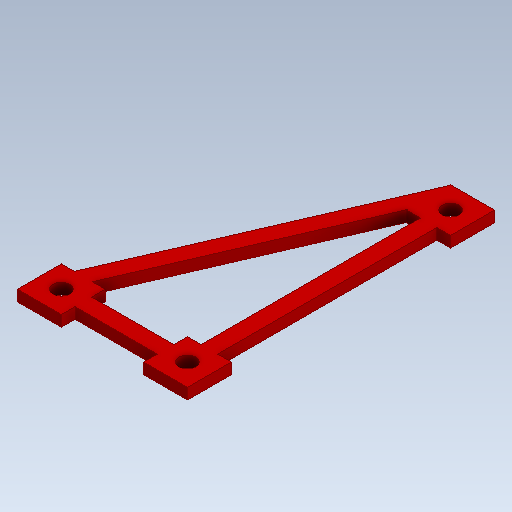
# Autodesk Inventor part: HexServoCoverV2
Saved by Autodesk Inventor 2020 (Build 240168000, 168)
## iProperties
Created: 2023-12-31
Part Number: HexServoCoverV2
Material: PETG
Document SubType Name: Modeling
Designer: smz3rm
Density: 1 g/cm^3
Appearance: Generic
Author: smz3rm
Autodesk Inventor part; units mm, degrees
ref_plane "YZ Plane" through (0, 0, 0) normal (1, 0, 0) x (0, 1, 0)
ref_plane "XZ Plane" through (0, 0, 0) normal (0, 1, 0) x (-1, 0, 0)
ref_plane "XY Plane" through (0, 0, 0) normal (0, 0, 1) x (1, 0, 0)
derived "HexBodyV2.ipt"
sketch "Sketch14" plane through (-59, -12, 62.4426) normal (0, 1, 0) x (1, 0, 0)
  line L0 (7, 63.7574) -> (48, 63.7574)
  line L1 (48, 63.7574) -> (48, 23.7574)
  line L2 (48, 23.7574) -> (7, 23.7574)
  line L3 (7, 23.7574) -> (7, 63.7574)
  line L4 (51, 66.7574) -> (4.5, 66.7574)
  line L5 (4.5, 20.7574) -> (51, 20.7574)
  line L6 (51, 20.7574) -> (51, 66.7574)
  line L7 (40, 66.7574) -> (40, 20.7574)
  line L8 (35, 66.7574) -> (35, 20.7574)
  line L9 (7, 63.7574) -> (35, 63.7574)
  line L10 (4, 43.7574) -> (51, 43.7574)
  line L11 (15.5, 66.7574) -> (15.5, 63.7574)
  line L12 (11, 66.7574) -> (11, 63.7574)
  line L13 (48, 53.7574) -> (54, 53.7574)
  line L14 (54, 53.7574) -> (59, 53.7574)
  line L15 (59, 167.4426) -> (59, -42.5574)
  line L16 (48, 68.5926) -> (48, 66.2926)
  line L17 (4.5, 66.7574) -> (4, 66.7574)
  line L18 (4, 8.833) -> (4, 87.1926)
  line L19 (4, 0.833) -> (4, 124.0523)
  line L20 (4.5, 20.7574) -> (4, 20.7574)
  line L21 (35, 23.7574) -> (27, 23.7574)
  line L22 (27, 23.7574) -> (27, 15.7574)
  line L23 (27, 15.7574) -> (35, 15.7574)
  line L24 (35, 15.7574) -> (35, 23.7574)
  line L25 (27, 63.7574) -> (27, 71.7574)
  line L26 (27, 71.7574) -> (35, 71.7574)
  line L27 (35, 71.7574) -> (35, 63.7574)
  line L28 (12, 23.7574) -> (4, 23.7574)
  line L29 (4, 23.7574) -> (4, 15.7574)
  line L30 (4, 15.7574) -> (12, 15.7574)
  line L31 (12, 15.7574) -> (12, 23.7574)
  line L32 (42, 63.8053) -> (42, 88.0017)
  line L33 (42, 66.7574) -> (42, 63.7574)
  line L34 (48, 63.7574) -> (48, 63.8053)
  line L35 (48, 63.8053) -> (42, 63.8053)
  line L36 (48, 63.7574) -> (48, 63.7574)
  line L37 (48, 63.7574) -> (48, 63.8053)
  point P0 (59, 62.4426)
  point P1 (34.5, 20.5208)
  point P2 (41, 65.8053)
  point P3 (11, 63.7574)
  point P4 (15.5, 63.7574)
  point P5 (48, 67.4426)
  point P6 (48, 43.7574)
  point P7 (40, 23.7574)
  point P8 (27, 66.7574)
  point P9 (35, 66.7574)
  point P10 (35, 20.7574)
  point P11 (27, 20.7574)
  point P12 (12, 20.7574)
  point P13 (40, 63.7574)
  point P14 (42, 63.8053)
  point P15 (42, 63.8053)
sketch "Sketch2" plane through (0, 0, 0) normal (0, 1, 0) x (-1, 0, 0)
  line L0 (32, -1.3148) -> (32, -9.3148) projected
  line L1 (32, -9.3148) -> (24, -9.3148) projected
  line L2 (24, -9.3148) -> (24, -1.3148) projected
  line L3 (32, 38.6852) -> (32, 46.6852) projected
  line L4 (24, 46.6852) -> (24, 38.6852) projected
  line L5 (32, 46.6852) -> (24, 46.6852) projected
  line L6 (55, 46.6852) -> (47, 46.6852) projected
  line L7 (47, 46.6852) -> (47, 38.6852) projected
  line L8 (47, 38.6852) -> (55, 38.6852) projected
  line L9 (55, 38.6852) -> (55, 46.6852)
  line L10 (32, 38.6852) -> (24, 38.6852)
  line L11 (32, -1.3148) -> (24, -1.3148)
  line L12 (32, -9.3148) -> (24, -1.3148)
  line L13 (32, 38.6852) -> (24, 46.6852)
  line L14 (55, 38.6852) -> (47, 46.6852)
  circle A0 centre (28, -5.3148) radius 1.55
  circle A1 centre (28, 42.6852) radius 1.55
  circle A2 centre (51, 42.6852) radius 1.55
  line L15 (47, 41.1852) -> (32, 41.1852)
  line L16 (32, 41.1852) -> (32, 44.1852)
  line L17 (32, 44.1852) -> (47, 44.1852)
  line L18 (47, 44.1852) -> (47, 41.1852)
  line L19 (29.5, -1.3148) -> (26.5, -1.3148)
  line L20 (26.5, -1.3148) -> (26.5, 38.6852)
  line L21 (26.5, 38.6852) -> (29.5, 38.6852)
  line L22 (29.5, 38.6852) -> (29.5, -1.3148)
  line L23 (51, 38.6852) -> (32, -5.3148)
  line L24 (32, -9.0985) -> (52.6339, 38.6852)
  line L25 (29.2458, -7.9092) -> (49.8797, 39.8745)
  point P0 (0, 0)
  point P1 (32, 42.6852)
  point P2 (47, 42.6852)
  point P3 (28, 38.6852)
  point P4 (49.3661, 38.6852)
  point P5 (32, -1.5311)
  point P6 (29.5, 38.6852)
  point P7 (47, 44.1852)
  point P8 (26.5, 38.6852)
  point P9 (26.5, -1.3148)
  dimension "d1" = 3.1
  dimension "d2" = 3.1
  dimension "d3" = 3.1
  dimension "d4" = 3
  dimension "d5" = 3
  dimension "d6" = 3
  constraints: 34 end point, 11 midpoint, 8 parallel, 4 perpendicular, 4 point on line, 3 centre point, 2 horizontal, 2 symmetric about line
  measures "d1" diameter of A0
  measures "d2" diameter of A1
  measures "d3" diameter of A2
  measures "d4" distance between parallel lines of L17 L15
  measures "d5" distance between parallel lines of L20 L22
  measures "d6" distance between parallel lines of L25 L24
extrude "Extrusion1" add sketch "Sketch2" along normal blind 2 contours L23 L8 L24 L0 | L0 L12 L25 | L0 L25 L8 L23 | L25 L12 A0 L11 L0 | L8 L7 L14 A2 | L1 L2 L12 A0 | L14 A2 L6 L9 | L11 L20 L10 L22 | L10 L4 L13 A1 | L15 L3 L17 L7 | L13 A1 L5 L3
equation "\"d1\" = M3ScrewDia"
equation "\"d2\" = M3ScrewDia"
equation "\"d3\" = M3ScrewDia"
equation "\"d5\" = d4"
equation "\"d6\" = d5"
equation "\"M3ScrewDia\" = 3.1"
body "Solid1"
